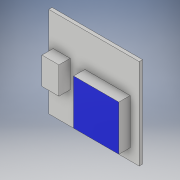
# Autodesk Inventor part: oledlcd
Saved by Autodesk Inventor 2019 (Build 230136000, 136)
## iProperties
Created: 2018-06-16
Part Number: oledlcd
Material: Generic
Document SubType Name: Modeling
Designer: daniel
Density: 1 g/cm^3
Appearance: Default
Author: daniel
Autodesk Inventor part; units mm, degrees
ref_plane "YZ Plane" through (0, 0, 0) normal (1, 0, 0) x (0, 1, 0)
ref_plane "XZ Plane" through (0, 0, 0) normal (0, 1, 0) x (-1, 0, 0)
ref_plane "XY Plane" through (0, 0, 0) normal (0, 0, 1) x (1, 0, 0)
sketch "Sketch1" plane through (0, 0, 0) normal (0, 0, 1) x (1, 0, 0)
  line L0 (-20, -20) -> (20, -20)
  line L1 (20, -20) -> (20, 20)
  line L2 (20, 20) -> (-20, 20)
  line L3 (-20, 20) -> (-20, -20)
  line L4 (-20, -20) -> (20, 20) construction
  line L5 (20, -20) -> (-20, 20) construction
  point P0 (0, 0)
  dimension "d0" = 40
  dimension "d1" = 40
  constraints: 12 end point, 2 midpoint, 2 parallel, 1 horizontal, 1 perpendicular
  measures "d0" distance of L2.end L1.end
  measures "d1" distance of L1.end L0.end
extrude "Extrusion1" add sketch "Sketch1" along normal blind 1.5
sketch "Sketch2" plane through (0, 0, 1.5) normal (0, 0, 1) x (1, 0, 0)
  line L0 (-28, 0) -> (28, 0) projected
  line L1 (-18, -6) -> (-10.5, -6)
  line L2 (-10.5, -6) -> (-10.5, 6)
  line L3 (-10.5, 6) -> (-18, 6)
  line L4 (-18, 6) -> (-18, -6)
  line L5 (-18, -6) -> (-10.5, 6) construction
  line L6 (-10.5, -6) -> (-18, 6) construction
  line L7 (-20, 20) -> (-20, -20) projected
  point P0 (0, 0)
  point P1 (-14.25, 0)
  dimension "d4" = 7.5
  dimension "d5" = 12
  dimension "d6" = 2
  constraints: 12 end point, 2 midpoint, 2 parallel, 1 horizontal, 1 perpendicular, 1 point on line
  measures "d4" distance of L3.end L2.end
  measures "d5" distance of L2.end L1.end
  measures "d6" distance between parallel lines of L7 L4
extrude "Extrusion2" add sketch "Sketch2" along normal blind 5
sketch "Sketch3" plane through (0, 0, 1.5) normal (0, 0, 1) x (1, 0, 0)
  line L0 (16, -15) -> (-4, -15)
  line L1 (-4, -15) -> (-4, 5)
  line L2 (-4, 5) -> (16, 5)
  line L3 (16, 5) -> (16, -15)
  line L4 (20, -20) -> (20, 20) projected
  line L5 (-20, -20) -> (20, -20) projected
  point P0 (0, 0)
  dimension "d9" = 4
  dimension "d10" = 5
  dimension "d11" = 20
  dimension "d12" = 20
  constraints: 8 end point, 2 parallel, 1 horizontal, 1 perpendicular
  measures "d9" distance between parallel lines of L3 L4
  measures "d10" distance between parallel lines of L5 L0
  measures "d11" distance of L2.end L0.start
  measures "d12" distance of L1.end L2.end
extrude "Extrusion3" add sketch "Sketch3" along normal blind 5
body "Solid1"
